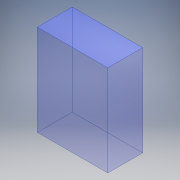
# Autodesk Inventor part: add
Saved by Autodesk Inventor 2018.1 (Build 221171000, 171)
## iProperties
Created: 2017-10-13
Part Number: add
Material: 一般
Document SubType Name: Modeling
Designer: kuwano
Density: 1 g/cm^3
Appearance: クリア - 青
Author: kuwano
Autodesk Inventor part; units mm, degrees
ref_plane "YZ Plane" through (0, 0, 0) normal (1, 0, 0) x (0, 1, 0)
ref_plane "XZ Plane" through (0, 0, 0) normal (0, 1, 0) x (-1, 0, 0)
ref_plane "XY Plane" through (0, 0, 0) normal (0, 0, 1) x (1, 0, 0)
sketch "スケッチ1" plane through (0, 0, 0) normal (0, 1, 0) x (-1, 0, 0)
  line L0 (341.5, 441.624) -> (-341.5, 441.624)
  line L1 (-341.5, 441.624) -> (-341.5, -441.624)
  line L2 (-341.5, -441.624) -> (341.5, -441.624)
  line L3 (341.5, -441.624) -> (341.5, 441.624)
  line L4 (0, -618.2736) -> (0, 618.2736) projected
  line L5 (478.1, 0) -> (-478.1, 0) projected
  point P0 (0, 0)
  point P1 (0, 441.624)
  point P2 (341.5, 0)
  dimension "d0" = 883.248
  dimension "d1" = 683
  constraints: 8 end point, 2 midpoint, 2 parallel, 2 point on line, 1 horizontal, 1 perpendicular
  measures "d0" distance of L2.end L0.start
  measures "d1" distance of L0.start L0.end
extrude "押し出し1" add sketch "スケッチ1" along normal blind 338.552
